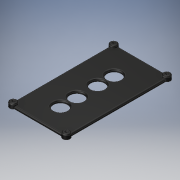
# Autodesk Inventor part: Case Top
Saved by Autodesk Inventor 2017 (Build 210142000, 142)
## iProperties
Created: 2018-01-14
Part Number: Case Top
Material: Generic
Document SubType Name: Modeling
Designer: Mitch
Density: 1 g/cm^3
Appearance: Glossy - Black
Author: Mitch
Autodesk Inventor part; units mm, degrees
ref_plane "YZ Plane" through (0, 0, 0) normal (1, 0, 0) x (0, 1, 0)
ref_plane "XZ Plane" through (0, 0, 0) normal (0, 1, 0) x (-1, 0, 0)
ref_plane "XY Plane" through (0, 0, 0) normal (0, 0, 1) x (1, 0, 0)
sketch "Sketch1" plane through (0, 0, 0) normal (0, 1, 0) x (-1, 0, 0)
  line L0 (0, 0) -> (76.2, 0)
  line L1 (76.2, 0) -> (76.2, -139.7)
  line L2 (76.2, -139.7) -> (0, -139.7)
  line L3 (0, -139.7) -> (0, 0)
  dimension "d0" = 76.2
  dimension "d1" = 139.7
  constraints: 8 end point, 2 parallel, 1 horizontal, 1 perpendicular
  measures "d0" distance of L1.end L2.end
  measures "d1" distance of L0.end L1.end
extrude "Extrusion1" add sketch "Sketch1" along normal blind 3.175
sketch "Sketch2" plane through (0, 3.175, 0) normal (0, 1, 0) x (1, 0, 0)
  line L0 (-76.2, 0) -> (0, 0) projected
  line L1 (0, 0) -> (0, 139.7) projected
  line L2 (0, 139.7) -> (-76.2, 139.7) projected
  line L3 (-76.2, 139.7) -> (-76.2, 0) projected
  circle A0 centre (-2.3876, 2.3876) radius 4.7625
  circle A1 centre (-73.8124, 2.3876) radius 4.7625
  circle A2 centre (-73.8124, 137.3124) radius 4.7625
  circle A3 centre (-2.3876, 137.3124) radius 4.7625
  dimension "d4" = 9.525
  dimension "d5" = 9.525
  dimension "d6" = 9.525
  dimension "d7" = 9.525
  dimension "d8" = 2.3876
  dimension "d9" = 2.3876
  dimension "d10" = 2.3876
  dimension "d11" = 2.3876
  dimension "d12" = 2.3876
  dimension "d13" = 2.3876
  dimension "d14" = 2.3876
  dimension "d15" = 2.3876
  constraints: 4 centre point
  measures "d4" diameter of A0
  measures "d5" diameter of A1
  measures "d6" diameter of A2
  measures "d7" diameter of A3
  measures "d8" distance from line of L0 A1.centre
  measures "d9" distance from line of L3 A1.centre
  measures "d10" distance from line of L1 A0.centre
  measures "d11" distance from line of L0 A0.centre
  measures "d12" distance from line of L2 A3.centre
  measures "d13" distance from line of L1 A3.centre
  measures "d14" distance from line of L2 A2.centre
  measures "d15" distance from line of L3 A2.centre
extrude "Extrusion2" add sketch "Sketch2" along normal mid plane 6.35 contours L3 A1 L0 | L0 A1 L3 | A0 L1 L0 | L0 L1 A0 | A2 L2 L3 | L3 L2 A2 | A3 L2 L1 | L1 L2 A3
fillet "Fillet1" radius 1.5875 4 edges at (-78.5749, 6.35, -2.3876) (-7.1501, 6.35, -2.3876) (-7.1501, 6.35, -137.3124) (-78.5749, 6.35, -137.3124)
hole "Hole1" at (-73.8124, 6.35, -2.3876) direction (0, -1, 0) diameter 2.4384 end through all countersink diameter 4.3688 countersink angle 82 clearance for "Flat Head Machine Screw (82)" size "#2" standard "Ansi Unified Screw Threads"
hole "Hole2" at (-73.8124, 6.35, -137.3124) direction (0, -1, 0) diameter 2.4384 end through all countersink diameter 4.3688 countersink angle 82 clearance for "Flat Head Machine Screw (82)" size "#2" standard "Ansi Unified Screw Threads"
hole "Hole3" at (-2.3876, 6.35, -137.3124) direction (0, -1, 0) diameter 2.4384 end through all countersink diameter 4.3688 countersink angle 82 clearance for "Flat Head Machine Screw (82)" size "#2" standard "Ansi Unified Screw Threads"
hole "Hole4" at (-2.3876, 6.35, -2.3876) direction (0, -1, 0) diameter 2.4384 end through all countersink diameter 4.3688 countersink angle 82 clearance for "Flat Head Machine Screw (82)" size "#2" standard "Ansi Unified Screw Threads"
sketch "Sketch5" plane through (0, 3.175, 0) normal (0, 1, 0) x (1, 0, 0)
  circle A0 centre (-39.2303, 31.2484) radius 8.9535 projected
  circle A1 centre (-39.2303, 53.3464) radius 8.9535 projected
  circle A2 centre (-39.2303, 81.2864) radius 8.9535 projected
  circle A3 centre (-39.2303, 103.3844) radius 8.9535 projected
  circle A4 centre (-39.2303, 31.2484) radius 9.4615
  circle A5 centre (-39.2303, 53.3464) radius 9.4615
  circle A6 centre (-39.2303, 81.2864) radius 9.4615
  circle A7 centre (-39.2303, 103.3844) radius 9.4615
  point P0 (0, 0)
  dimension "d67" = 0.508
  dimension "d68" = 0.508
  dimension "d69" = 0.508
  dimension "d70" = 0.508
  constraints: 4 centre point
  measures "d67" radial gap between concentric circles of A0 A4
  measures "d68" radial gap between concentric circles of A1 A5
  measures "d69" radial gap between concentric circles of A2 A6
  measures "d70" radial gap between concentric circles of A3 A7
extrude "Extrusion5" cut sketch "Sketch5" against normal blind 6.35 contours A0 | A1 | A2 | A3 | A4 | A5 | A6 | A7
fillet "Fillet2" radius 1.5875 4 edges at (-48.6918, 3.175, -31.2484) (-48.6918, 3.175, -53.3464) (-48.6918, 3.175, -81.2864) (-48.6918, 3.175, -103.3844)
fillet "Fillet3" radius 1.5875 4 edges at (-38.1, 3.175, 0) (0, 3.175, -69.85) (-76.2, 3.175, -69.85) (-38.1, 3.175, -139.7)
body "Solid1"
